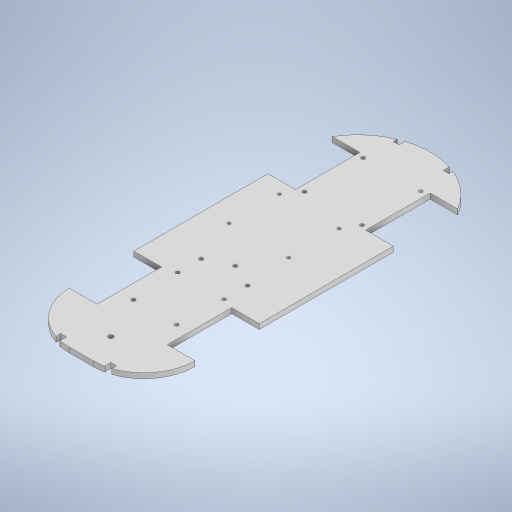
# Autodesk Inventor part: base automodel
Saved by Autodesk Inventor 2024 (Build 280153000, 153)
## iProperties
Created: 2023-10-17
Part Number: base automodel
Material: Generic
Document SubType Name: Modeling
Designer: dm1303
Density: 1 g/cm^3
Appearance: Default
Author: dm1303
Autodesk Inventor part; units mm, degrees
ref_plane "YZ Plane" through (0, 0, 0) normal (1, 0, 0) x (0, 1, 0)
ref_plane "XZ Plane" through (0, 0, 0) normal (0, 1, 0) x (-1, 0, 0)
ref_plane "XY Plane" through (0, 0, 0) normal (0, 0, 1) x (1, 0, 0)
sketch "Sketch1" plane through (0, 0, 0) normal (0, 1, 0) x (-1, 0, 0)
  line L0 (-11.6621, 194.9999) -> (11.3379, 194.9999)
  line L1 (60.8379, 145.4999) -> (60.8379, -109.9001)
  line L2 (-61.1621, -109.9001) -> (-61.1621, 145.4999)
  line L3 (-61.1621, 194.9999) -> (61.1621, -194.9999) construction
  line L4 (60.8379, 194.9999) -> (-60.8379, -194.9999) construction
  arc A0 (60.8379, 145.4999) -> (11.3379, 194.9999) centre (11.3379, 145.4999) ccw
  arc A1 (-11.6621, 194.9999) -> (-61.1621, 145.4999) centre (-11.6621, 145.4999) ccw
  line L5 (-61.1621, 145.4999) -> (-34.3621, 145.4999)
  line L6 (-34.3621, 145.4999) -> (-34.3621, 82.9999)
  line L7 (-34.3621, 82.9999) -> (-61.1621, 82.9999)
  line L8 (-61.1621, 82.9999) -> (-61.1621, 145.4999)
  line L9 (-61.1621, 82.9999) -> (-61.1621, -47.4001)
  line L10 (-61.1621, -47.4001) -> (-34.3621, -47.4001)
  line L11 (-34.3621, -47.4001) -> (-34.3621, -109.9001)
  line L12 (-34.3621, -109.9001) -> (-61.1621, -109.9001)
  line L13 (-61.1621, -109.9001) -> (-61.1621, -47.4001)
  line L14 (60.8379, 145.4999) -> (34.0379, 145.4999)
  line L15 (34.0379, 145.4999) -> (34.0379, 82.9999)
  line L16 (34.0379, 82.9999) -> (60.8379, 82.9999)
  line L17 (60.8379, 82.9999) -> (60.8379, 145.4999)
  line L18 (60.8379, -47.4001) -> (34.0379, -47.4001)
  line L19 (34.0379, -47.4001) -> (34.0379, -109.9001)
  line L20 (34.0379, -109.9001) -> (60.8379, -109.9001)
  line L21 (60.8379, -109.9001) -> (60.8379, -47.4001)
  arc A2 (-61.1621, -109.9001) -> (60.8379, -109.9001) centre (-0.1621, -73.7641) ccw
  point P0 (0, 0)
  dimension "d0" = 122
  dimension "d1" = 390
  dimension "d2" = 49.5
  dimension "d4" = 26.8
  dimension "d5" = 62.5
  dimension "d6" = 130.4
  dimension "d7" = 26.8
  dimension "d8" = 62.5
  dimension "d9" = 26.8
  dimension "d10" = 62.5
  dimension "d11" = 26.8
  dimension "d12" = 62.5
  dimension "d13" = 70.9
  constraints: 44 end point, 9 parallel, 6 point on circle, 6 point on line, 5 horizontal, 5 perpendicular, 4 tangent, 3 centre point, 2 midpoint, 1 equal radius
  measures "d0" distance of L3.end L4.end
  measures "d1" distance of L4.start L3.end
  measures "d2" radius of A0
  measures "d4" distance of L6.end L7.end
  measures "d5" distance of L5.end L6.end
  measures "d6" distance of L7.end L9.end
  measures "d7" distance of L2.start L11.end
  measures "d8" distance of L10.end L11.end
  measures "d9" distance of L16.end L15.end
  measures "d10" distance of L15.end L14.end
  measures "d11" distance of L1.end L19.end
  measures "d12" distance of L19.end L18.end
  measures "d13" radius of A2
extrude "Extrusion1" add sketch "Sketch1" along normal blind 5 contours L0 A0 L14 L15 L16 L1 L18 L19 L20 A2 L12 L11 L10 L2 L7 L6 L5 A1
sketch "Boceto2" plane through (0, 5, 0) normal (0, 1, 0) x (1, 0, 0)
  point P0 (0, 0)
sketch "Boceto3" plane through (0, 5, 0) normal (0, 1, 0) x (1, 0, 0)
  line L0 (-11.3379, -194.9999) -> (11.6621, -194.9999) projected
  line L1 (0.1621, -194.9999) -> (0.1621, -184.9999)
  line L2 (-2.7008, -183.6215) -> (19.0062, -183.6215)
  line L3 (19.0062, -183.6215) -> (-18.9938, -183.6215)
  line L4 (-2.7008, -148.6215) -> (19.0062, -148.6215)
  line L5 (19.0062, -148.6215) -> (-18.9938, -148.6215)
  line L6 (-18.9938, -148.6215) -> (-18.9938, -183.6215)
  line L7 (19.0062, -148.6215) -> (19.0062, -183.6215)
  line L8 (61.1621, -82.9999) -> (61.1621, 47.4001) projected
  line L9 (-60.8379, 47.4001) -> (-60.8379, -82.9999) projected
  line L10 (21.7666, -187.8715) -> (27.3666, -187.8715)
  line L11 (27.3666, -187.8715) -> (27.3666, -193.8715)
  line L12 (27.3666, -193.8715) -> (21.7666, -193.8715)
  line L13 (21.7666, -193.8715) -> (21.7666, -187.8715)
  line L14 (-11.3379, -194.9999) -> (-14.1379, -194.9999)
  arc A0 (-60.8379, -145.4999) -> (-11.3379, -194.9999) centre (-11.3379, -145.4999) ccw projected
  line L15 (-26.8363, -187.8801) -> (-21.2363, -187.8801)
  line L16 (-21.2363, -187.8801) -> (-21.2363, -193.8801)
  line L17 (-21.2363, -193.8801) -> (-26.8363, -193.8801)
  line L18 (-26.8363, -193.8801) -> (-26.8363, -187.8801)
  line L19 (21.7169, 135.4811) -> (27.3169, 135.4811)
  arc A1 (61.1621, 109.9001) -> (-60.8379, 109.9001) centre (0.1621, 73.7641) ccw projected
  line L20 (21.6786, 141.4811) -> (27.2786, 141.4811)
  line L21 (27.2786, 141.4811) -> (27.2786, 135.4811)
  line L22 (27.2786, 135.4811) -> (21.6786, 135.4811)
  line L23 (21.6786, 135.4811) -> (21.6786, 141.4811)
  line L24 (-26.9249, 141.4803) -> (-21.3249, 141.4803)
  line L25 (-21.3249, 141.4803) -> (-21.3249, 135.4803)
  line L26 (-21.3249, 135.4803) -> (-26.9249, 135.4803)
  line L27 (-26.9249, 135.4803) -> (-26.9249, 141.4803)
  line L28 (0.404, 144.7464) -> (0.404, -197.1126)
  line L29 (-34.0379, 47.4001) -> (-60.8379, 47.4001) projected
  line L30 (-60.8379, 47.4001) -> (-50.8379, 47.4001)
  line L31 (-41.5224, -16.7155) -> (-41.5224, 39.2845)
  line L32 (-41.5224, 39.2845) -> (43.4776, 39.2845)
  line L33 (43.4776, 39.2845) -> (43.4776, -16.7155)
  line L34 (43.4776, -16.7155) -> (-41.5224, -16.7155)
  line L35 (0.544, 11.7839) -> (0.544, 15.8925)
  line L36 (0.9776, 39.2845) -> (0.9776, -16.7155)
  line L37 (-21.3249, 141.4803) -> (21.6751, 141.4803)
  arc A2 (-60.8379, -145.4999) -> (-11.3379, -194.9999) centre (-11.3379, -145.4999) ccw projected
  line L38 (-34.0379, -82.9999) -> (-34.0379, -145.4999) projected
  line L39 (-21.2334, -193.8715) -> (-21.2169, -197.8147)
  line L40 (21.1268, -127.3043) -> (21.1268, -110.8043)
  line L41 (21.9297, -127.1387) -> (21.9297, -124.1387)
  line L42 (21.9297, -124.1387) -> (-19.9703, -124.1387)
  circle A3 centre (21.9297, -124.1387) radius 1.75
  circle A4 centre (-19.9703, -124.1387) radius 1.75
  line L43 (0.9797, -124.1387) -> (0.9776, -46.1387)
  circle A5 centre (0.9776, -46.1387) radius 1.75
  line L44 (3.2596, -48.0861) -> (0.432, -49.0887)
  line L45 (0.432, -49.0887) -> (-1.8499, -47.1412)
  line L46 (-1.8499, -47.1412) -> (-1.3044, -44.1913)
  line L47 (-1.3044, -44.1913) -> (1.5231, -43.1887)
  line L48 (1.5231, -43.1887) -> (3.8051, -45.1361)
  line L49 (3.8051, -45.1361) -> (3.2596, -48.0861)
  line L50 (0.9777, -49.2626) -> (28.4777, -49.2619)
  line L51 (28.4777, -49.2619) -> (-26.5223, -49.2619)
  line L52 (-26.5223, -49.2619) -> (-26.5223, -87.0619)
  line L53 (-26.5223, -87.0619) -> (28.4777, -87.0619)
  line L54 (28.4777, -87.0619) -> (28.4777, -49.2619)
  line L55 (-26.5223, -49.2619) -> (-23.3223, -49.2619)
  line L56 (-23.3223, -49.2619) -> (-23.3223, -54.9619)
  line L57 (-23.3223, -54.9619) -> (-21.5723, -54.9619)
  line L58 (-21.5723, -54.9619) -> (-21.5723, -56.7119)
  circle A6 centre (-21.5723, -56.7119) radius 1.75
  line L59 (-21.5723, -56.7119) -> (28.4777, -56.7119)
  line L60 (-21.5723, -56.7119) -> (-21.5723, -87.0619)
  line L61 (28.4777, -87.0619) -> (23.5277, -87.0619)
  line L62 (23.5277, -87.0619) -> (23.5277, -79.6119)
  circle A7 centre (23.5277, -79.6119) radius 1.75
  line L63 (23.5277, -79.6119) -> (-26.5223, -79.6119)
  line L64 (23.5277, -79.6119) -> (23.5277, -49.2619)
  circle A8 centre (23.5277, -56.7119) radius 1.75
  circle A9 centre (-21.5723, -79.6119) radius 1.75
  line L65 (-18.9938, -183.6215) -> (0.0062, -183.6215)
  line L66 (0.0062, -183.6215) -> (0.0062, -148.6215)
  line L67 (-21.2334, -193.8715) -> (21.7666, -193.8715)
  circle A10 centre (0.0062, -166.1215) radius 2.3
  line L68 (-41.5224, 39.2845) -> (-38.0224, 39.2845)
  line L69 (-38.0224, 39.2845) -> (-38.0224, 35.7845)
  line L70 (-38.0224, 35.7845) -> (19.9776, 35.7845)
  line L71 (19.9776, 35.7845) -> (19.9776, -13.2155)
  line L72 (19.9776, -13.2155) -> (-38.0224, -13.2155)
  line L73 (-38.0224, -13.2155) -> (-38.0224, 35.7845)
  circle A11 centre (-38.0224, 35.7845) radius 1.4
  circle A12 centre (19.9776, 35.7845) radius 1.4
  circle A13 centre (19.9776, -13.2155) radius 1.4
  circle A14 centre (-38.0224, -13.2155) radius 1.4
  line L74 (-34.0379, 109.9001) -> (-31.8379, 109.9001)
  line L75 (34.3621, 47.4001) -> (34.3621, 109.9001) projected
  line L76 (34.3621, 109.9001) -> (32.1621, 109.9001)
  line L77 (-31.8379, 109.9001) -> (32.1621, 109.9001)
  line L78 (32.1621, 109.9001) -> (32.1621, 47.4001)
  line L79 (32.1621, 47.4001) -> (-31.8379, 47.4001)
  line L80 (-31.8379, 47.4001) -> (-31.8379, 109.9001)
  line L81 (-31.8379, 109.9001) -> (-27.8379, 109.9001)
  line L82 (-27.8379, 109.9001) -> (-27.8379, 106.9001)
  line L83 (-27.8379, 106.9001) -> (28.1621, 106.9001)
  line L84 (28.1621, 106.9001) -> (28.1621, 49.9001)
  line L85 (28.1621, 49.9001) -> (-27.8379, 49.9001)
  line L86 (-27.8379, 49.9001) -> (-27.8379, 106.9001)
  circle A15 centre (-27.8379, 106.9001) radius 1.75
  circle A16 centre (28.1621, 106.9001) radius 1.75
  circle A17 centre (-27.8379, 49.9001) radius 1.75
  circle A18 centre (28.1621, 49.9001) radius 1.75
  point P0 (-21.5954, -147.627)
  point P1 (-17.4759, -197.9035)
  point P2 (-17.3346, -191.9653)
  point P3 (21.8949, -190.8298)
  point P4 (-20.3189, 140.8602)
  point P5 (0.404, -148.6215)
  point P6 (21.7169, 135.4811)
  point P7 (27.2786, 135.4811)
  point P8 (-26.8363, -192.5111)
  point P9 (-21.2363, -194.0001)
  point P10 (0.404, -148.6215)
  point P11 (-21.8071, -193.8801)
  point P12 (0.404, -183.6215)
  dimension "d16" = 10
  dimension "d18" = 38
  dimension "d19" = 35
  dimension "d21" = 38
  dimension "d29" = 5.6
  dimension "d30" = 6
  dimension "d36" = 5.6
  dimension "d44" = 5.6
  dimension "d45" = 6
  dimension "d46" = 5.6
  dimension "d47" = 6
  dimension "d69" = 56
  dimension "d70" = 85
  dimension "d128" = 16.5
  dimension "d133" = 3
  dimension "d134" = 3.5
  dimension "d135" = 3.5
  dimension "d136" = 78
  dimension "d137" = 41.9
  dimension "d138" = 3.5
  dimension "d139" = 3
  dimension "d140" = 27.5
  dimension "d141" = 55
  dimension "d142" = 37.8
  dimension "d143" = 3.2
  dimension "d144" = 5.7
  dimension "d146" = 1.75
  dimension "d147" = 1.75
  dimension "d148" = 3.5
  dimension "d149" = 4.95
  dimension "d150" = 7.45
  dimension "d151" = 3.5
  dimension "d152" = 3.5
  dimension "d153" = 3.5
  dimension "d156" = 19
  dimension "d157" = 35
  dimension "d158" = 90
  dimension "d159" = 43
  dimension "d160" = 43
  dimension "d161" = 4.6
  dimension "d164" = 3.5
  dimension "d165" = 3.5
  dimension "d166" = 58
  dimension "d167" = 49
  dimension "d168" = 58
  dimension "d169" = 90
  dimension "d170" = 2.8
  dimension "d171" = 2.8
  dimension "d172" = 2.8
  dimension "d173" = 2.8
  dimension "d174" = 2.2
  dimension "d175" = 2.2
  dimension "d176" = 62.5
  dimension "d177" = 64
  dimension "d178" = 4
  dimension "d179" = 3
  dimension "d180" = 56
  dimension "d181" = 57
  dimension "d182" = 3.5
  dimension "d183" = 3.5
  dimension "d184" = 3.5
  dimension "d185" = 3.5
  constraints: 162 end point, 24 perpendicular, 18 parallel, 18 point on line, 16 centre point, 14 coincident, 12 horizontal, 5 midpoint, 3 vertical, 1 tangent, 13 other
  measures "d16" distance of L1.start L1.end
  measures "d18" distance of L2.end L3.end
  measures "d19" distance of L2.start L4.start
  measures "d21" distance of L4.end L5.end
  measures "d29" distance of L11.end L12.end
  measures "d30" distance of L10.end L11.end
  measures "d36" distance of L16.end L17.end
  measures "d44" distance of L21.end L22.end
  measures "d45" distance of L20.end L21.end
  measures "d46" distance of L25.end L26.end
  measures "d47" distance of L24.end L25.end
  measures "d69" distance of L32.end L33.end
  measures "d70" distance of L31.end L32.end
  measures "d128" distance of L40.start L40.end
  measures "d133" distance of L41.start L41.end
  measures "d134" diameter of A3
  measures "d135" diameter of A4
  measures "d136" distance of L43.start L43.end
  measures "d137" distance of L41.end L42.end
  measures "d138" diameter of A5
  measures "d139" distance of L48.end L44.start
  measures "d140" distance of L50.start L50.end
  measures "d141" distance of L53.end L52.end
  measures "d142" distance of L52.end L51.end
  measures "d143" distance of L51.end L55.end
  measures "d144" distance of L55.end L56.end
  measures "d146" distance of L56.end L57.end
  measures "d147" distance of L57.end L58.end
  measures "d148" diameter of A6
  measures "d149" distance of L53.end L61.end
  measures "d150" distance of L61.end L62.end
  measures "d151" diameter of A7
  measures "d152" diameter of A8
  measures "d153" diameter of A9
  measures "d156" distance of L3.end L65.end
  measures "d157" distance of L65.end L66.end
  measures "d158" angle of L66 L65
  measures "d159" distance of L24.end L37.end
  measures "d160" distance of L39.start L12.end
  measures "d161" diameter of A10
  measures "d164" distance of L31.end L68.end
  measures "d165" distance of L68.end L69.end
  measures "d166" distance of L69.end L70.end
  measures "d167" distance of L70.end L71.end
  measures "d168" distance of L71.end L72.end
  measures "d169" angle of L71 L72
  measures "d170" diameter of A11
  measures "d171" diameter of A12
  measures "d172" diameter of A13
  measures "d173" diameter of A14
  measures "d174" distance of L74.start L74.end
  measures "d175" distance of L75.end L76.end
  measures "d176" distance of L77.end L78.end
  measures "d177" distance of L74.end L77.end
  measures "d178" distance of L74.end L81.end
  measures "d179" distance of L81.end L82.end
  measures "d180" distance of L82.end L83.end
  measures "d181" distance of L83.end L84.end
  measures "d182" diameter of A15
  measures "d183" diameter of A16
  measures "d184" diameter of A17
  measures "d185" diameter of A18
extrude "Extrusión2" add sketch "Boceto3" against normal blind 1 contours L2 L66 A10 L28 | L28 A10 L4 L7 L2 | L2 L3 L6 L5 L4 L66 A10 | A10 L66 L28 | L28 A10 | A10 L66 | A10 L66 L4 L28
extrude "Extrusión4" cut sketch "Boceto3" against normal blind 20 contours L17 L18 A0 | A0 L18 L15 L16 L17 | L23 L20 L21 A1 | A1 L21 L19 L22 L23 | L13 L10 L11 L12 | L25 L26 L27 A1 | A1 L27 L24 L25
extrude "Extrusión6" cut sketch "Boceto3" against normal blind 10 contours A14 L73 L72 | L72 L73 A14 | A11 L73 L70 | L70 L69 A11 | A13 L71 L72 | L72 L71 A13 | L73 A11 L69 | A12 L71 L70 | L70 L71 A12
extrude "Extrusión7" cut sketch "Boceto3" against normal blind 5 contours A4 | A3 L40 L42 | L42 L40 A3 | A9 L60 L63 | L63 L60 A9 | A9 L63 L60 | L42 L41 A3 L40 | L40 A3 L41 L42 | L59 L58 A6 | A6 L60 L59 | L63 L62 A7 | A7 L64 L63 | L63 A9 L60 | L62 L64 A7 | L58 L60 A6 | A8 L64 L59 | L59 L64 A8 | A5 L28 | L28 A5 | L64 A8 L59 | L59 A8 L64
extrude "Extrusión8" cut sketch "Boceto3" against normal blind 5 contours A10 L66 L28 | L28 A10 | A10 L66
extrude "Extrusión9" cut sketch "Boceto3" against normal blind 10 contours A18 L84 L85 | L85 L84 A18 | A17 L86 L85 | L85 L86 A17 | A15 L86 L83 | L83 L82 A15 | A16 L84 L83 | L83 L84 A16 | L86 A15 L82
body "Solid1"
